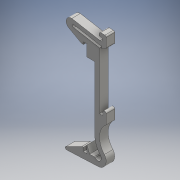
# Autodesk Inventor part: raspDinClipmmv4
Saved by Autodesk Inventor 2016 (Build 200138000, 138)
## iProperties
Created: 2016-08-27
Part Number: raspDinClipmmv4
Material: Generic
Document SubType Name: Modeling
Designer: Thetheos
Density: 1 g/cm^3
Appearance: Default
Author: Thetheos
Autodesk Inventor part; units mm, degrees
ref_plane "YZ Plane" through (0, 0, 0) normal (1, 0, 0) x (0, 1, 0)
ref_plane "XZ Plane" through (0, 0, 0) normal (0, 1, 0) x (-1, 0, 0)
ref_plane "XY Plane" through (0, 0, 0) normal (0, 0, 1) x (1, 0, 0)
sketch "Sketch1" plane through (0, 0, 0) normal (0, 1, 0) x (-1, 0, 0)
  arc A0 (-159.7794, 702.6597) -> (-160.5669, 701.8721) centre (-159.7794, 701.8721) ccw
  line L0 (-155.7462, 702.6597) -> (-155.7462, 704.2667)
  line L1 (-155.7462, 704.2667) -> (-153.5139, 704.2667)
  line L2 (-153.5139, 704.2667) -> (-153.5139, 702.7873)
  line L3 (-153.5139, 702.7873) -> (-152.617, 702.7873)
  arc A1 (-164.1836, 648.4268) -> (-160.5669, 657.8731) centre (-174.7114, 657.8731) ccw
  line L4 (-160.5669, 657.8731) -> (-160.5669, 701.8721)
  arc A2 (-160.1794, 645.8656) -> (-160.7583, 645.6139) centre (-160.1783, 645.0714) ccw
  arc A3 (-164.1836, 648.4268) -> (-160.7583, 645.6139) centre (-162.4137, 647.0901) ccw
  line L5 (-155.7462, 648) -> (-155.7462, 645.3343)
  line L6 (-155.7462, 645.3343) -> (-153.4959, 645.3343)
  line L7 (-153.4959, 645.3343) -> (-153.4959, 647.6194)
  arc A4 (-143.0505, 641.0266) -> (-142.8499, 642.7649) centre (-143.1474, 641.9185) ccw
  line L8 (-163.0481, 641.9081) -> (-143.0505, 641.0266)
  arc A5 (-166.527, 650.2868) -> (-163.0481, 641.9081) centre (-162.4027, 647.0877) ccw
  arc A6 (-166.527, 650.2868) -> (-167.6435, 666.7468) centre (-174.834, 657.9912) ccw
  arc A7 (-163.8545, 670.6656) -> (-163.5889, 670.9316) centre (-163.8582, 670.9349) ccw
  line L9 (-163.5889, 706.0242) -> (-163.5889, 706.0613)
  line L10 (-163.5889, 706.0613) -> (-147.5669, 708.9022)
  arc A8 (-147.5669, 708.9022) -> (-147.8202, 710.4852) centre (-147.6004, 709.7086) ccw
  line L11 (-147.8202, 710.4852) -> (-163.5831, 707.6952)
  line L12 (-163.5831, 707.6952) -> (-164.9831, 707.6944)
  line L13 (-164.9831, 707.6944) -> (-164.9826, 706.5463)
  arc A9 (-165.396, 706.3271) -> (-164.9826, 706.5463) centre (-165.2521, 706.5552) ccw
  line L14 (-165.396, 706.3271) -> (-167.2486, 707.3943)
  arc A10 (-167.6628, 708.0983) -> (-167.2486, 707.3943) centre (-166.8615, 708.0959) ccw
  line L15 (-167.6628, 708.0983) -> (-167.6658, 713.6939)
  arc A11 (-166.8627, 714.4991) -> (-167.6658, 713.6939) centre (-166.8611, 713.6943) ccw
  line L16 (-166.8627, 714.4991) -> (-164.1837, 714.5007)
  arc A12 (-163.3795, 713.6976) -> (-164.1837, 714.5007) centre (-164.1848, 713.6954) ccw
  line L17 (-163.3795, 713.6976) -> (-163.3787, 712.3581)
  line L18 (-163.3787, 712.3581) -> (-165.5216, 711.9789)
  line L19 (-165.5216, 711.9789) -> (-165.5215, 711.7106)
  arc A13 (-165.5215, 711.7106) -> (-163.8456, 710.1095) centre (-163.9177, 711.7116) ccw
  line L20 (-163.8456, 710.1095) -> (-146.318, 713.1891)
  arc A14 (-144.6103, 707.1134) -> (-146.318, 713.1891) centre (-146.0422, 709.9888) ccw
  arc A15 (-152.617, 702.7873) -> (-152.2474, 702.8795) centre (-152.6236, 703.6003) ccw
  line L21 (-155.7462, 702.6597) -> (-155.7462, 700.1597)
  line L22 (-155.7462, 700.1597) -> (-156.9462, 700.1597)
  line L23 (-156.9462, 700.1597) -> (-157.7628, 702.6597)
  line L24 (-157.7628, 702.6597) -> (-159.7794, 702.6597)
  line L25 (-155.7462, 648) -> (-155.7462, 650)
  line L26 (-155.7462, 650) -> (-157.3545, 645.8656)
  line L27 (-157.3545, 645.8656) -> (-160.1794, 645.8656)
  line L28 (-144.6103, 707.1134) -> (-152.2474, 702.8795)
  line L29 (-152.5619, 647.6194) -> (-153.4959, 647.6194)
  line L30 (-163.8545, 670.6656) -> (-165.2545, 670.6656)
  arc A16 (-165.4084, 670.8401) -> (-165.2545, 670.6656) centre (-165.2322, 670.8403) ccw
  line L31 (-163.5889, 670.9316) -> (-163.5889, 706.0613)
  line L32 (-165.4084, 670.8401) -> (-165.7258, 673.0171)
  line L33 (-167.6435, 666.7468) -> (-167.6435, 672.6833)
  line L34 (-142.8499, 642.7649) -> (-152.5619, 647.6194)
  arc A17 (-165.7258, 673.0171) -> (-167.6435, 672.6833) centre (-166.6444, 672.619) ccw
  point P0 (-160.5669, 683.588)
  dimension "d2" = 43.999
  dimension "d6" = 2.5
  dimension "d7" = 1.2
  dimension "d8" = 2
  dimension "d18" = 1.4
  dimension "d20" = 2.2
  dimension "d21" = 1.4
  dimension "d22" = 4.0546
  constraints: 70 end point, 36 point on circle, 18 centre point, 6 perpendicular, 4 horizontal, 2 vertical, 1 parallel, 1 tangent
  measures "d2" distance of L4.start L4.end
  measures "d6" distance of L0.start L21.end
  measures "d7" distance of L21.end L22.end
  measures "d8" distance of L5.start L25.end
  measures "d18" distance of L30.start L30.end
  measures "d20" distance of L32.start L32.end
  measures "d21" distance of L12.start L12.end
  measures "d22" distance between parallel lines of L33 L31
extrude "Extrusion1" add sketch "Sketch1" along normal blind 5.3
sketch "Sketch2" plane through (0, 0, 0) normal (0, -1, 0) x (1, 0, 0)
  line L0 (156.9462, 700.1597) -> (155.7462, 700.1597) projected
  line L1 (155.7462, 700.1597) -> (155.7462, 697.1597)
  line L2 (155.7462, 697.1597) -> (160.5669, 697.1597)
  line L3 (160.5669, 657.8731) -> (160.5669, 701.8721) projected
  line L4 (160.5669, 697.1597) -> (160.5783, 702.6397)
  line L5 (160.5783, 702.6397) -> (155.7462, 704.198)
  line L6 (155.7462, 704.198) -> (155.7462, 700.1597)
  point P0 (0, 0)
  dimension "d9" = 3
  constraints: 10 end point, 1 collinear, 1 perpendicular, 1 point on line, 1 vertical
  measures "d9" distance of L0.end L1.end
extrude "Extrusion2" add sketch "Sketch2" against normal blind 5.3
sketch "Sketch3" plane through (155.7462, 0, 704.2667) normal (-1, 0, 0) x (0, 0, 1)
  circle A0 centre (-4.5576, 2.65) radius 1.25
  line L0 (-7.107, 5.3) -> (0, 5.3) projected
  line L1 (0, 0) -> (-7.107, 0) projected
  point P0 (-704.2667, 0)
  dimension "d12" = 2.5
  dimension "d14" = 2.65
  dimension "d15" = 2.65
  constraints: 1 centre point
  measures "d12" diameter of A0
  measures "d14" distance from line of A0.centre L0
  measures "d15" distance from line of L1 A0.centre
extrude "Extrusion3" cut sketch "Sketch3" against normal blind 5
body "Solid1"
